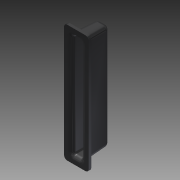
# Autodesk Inventor part: rubber-chamber
Saved by Autodesk Inventor 2015 (Build 190159000, 159)
## iProperties
Created: 2014-10-09
Part Number: rubber-chamber
Material: Rubber
Document SubType Name: Modeling
Designer: Adam
Density: 0.93 g/cm^3
Appearance: Rubber - Black - Version 1.1
Author: Adam
Autodesk Inventor part; units mm, degrees
ref_plane "YZ Plane" through (0, 0, 0) normal (1, 0, 0) x (0, 1, 0)
ref_plane "XZ Plane" through (0, 0, 0) normal (0, 1, 0) x (-1, 0, 0)
ref_plane "XY Plane" through (0, 0, 0) normal (0, 0, 1) x (1, 0, 0)
ref_plane "Work Plane1" through (0, 0, 0) normal (0, 0, 1) x (1, 0, 0)
sketch "Sketch1" plane through (0, 0, 0) normal (0, 0, 1) x (1, 0, 0)
  arc A0 (-28.0193, -5.5) -> (-30.0193, -3.5) centre (-30.0193, -5.5) ccw projected
  line L0 (-40.0193, -3.5) -> (-30.0193, -3.5) projected
  arc A1 (-40.0193, -3.5) -> (-42.0193, -5.5) centre (-40.0193, -5.5) ccw projected
  line L1 (-42.0193, -66.5) -> (-42.0193, -5.5) projected
  arc A2 (-42.0193, -66.5) -> (-40.0193, -68.5) centre (-40.0193, -66.5) ccw projected
  line L2 (-40.0193, -68.5) -> (-30.0193, -68.5) projected
  arc A3 (-30.0193, -68.5) -> (-28.0193, -66.5) centre (-30.0193, -66.5) ccw projected
  line L3 (-28.0193, -66.5) -> (-28.0193, -5.5) projected
  line L4 (-30.5193, -7.5) -> (-30.5193, -64.5) projected
  arc A4 (-32.0193, -66) -> (-30.5193, -64.5) centre (-32.0193, -64.5) ccw projected
  line L5 (-32.0193, -66) -> (-38.0193, -66) projected
  arc A5 (-39.5193, -64.5) -> (-38.0193, -66) centre (-38.0193, -64.5) ccw projected
  line L6 (-39.5193, -64.5) -> (-39.5193, -7.5) projected
  arc A6 (-38.0193, -6) -> (-39.5193, -7.5) centre (-38.0193, -7.5) ccw projected
  line L7 (-38.0193, -6) -> (-32.0193, -6) projected
  arc A7 (-30.5193, -7.5) -> (-32.0193, -6) centre (-32.0193, -7.5) ccw projected
  arc A8 (-28.3193, -5.5) -> (-30.0193, -3.8) centre (-30.0193, -5.5) ccw
  arc A9 (-40.0193, -3.8) -> (-41.7193, -5.5) centre (-40.0193, -5.5) ccw
  line L8 (-30.0193, -3.8) -> (-40.0193, -3.8)
  arc A10 (-30.0193, -68.2) -> (-28.3193, -66.5) centre (-30.0193, -66.5) ccw
  line L9 (-28.3193, -5.5) -> (-28.3193, -66.5)
  line L10 (-30.0193, -68.2) -> (-40.0193, -68.2)
  line L11 (-41.7193, -5.5) -> (-41.7193, -66.5)
  arc A11 (-41.7193, -66.5) -> (-40.0193, -68.2) centre (-40.0193, -66.5) ccw
  arc A12 (-31.0193, -7.5) -> (-32.0193, -6.5) centre (-32.0193, -7.5) ccw
  arc A13 (-38.0193, -6.5) -> (-39.0193, -7.5) centre (-38.0193, -7.5) ccw
  arc A14 (-32.0193, -65.5) -> (-31.0193, -64.5) centre (-32.0193, -64.5) ccw
  arc A15 (-39.0193, -64.5) -> (-38.0193, -65.5) centre (-38.0193, -64.5) ccw
  line L12 (-32.0193, -65.5) -> (-38.0193, -65.5)
  line L13 (-32.0193, -6.5) -> (-38.0193, -6.5)
  line L14 (-39.0193, -7.5) -> (-39.0193, -64.5)
  line L15 (-31.0193, -7.5) -> (-31.0193, -64.5)
  point P0 (0, 0)
  dimension "d0" = 0.3
  dimension "d1" = 0.5
  constraints: 17 point on circle, 16 end point, 14 tangent, 8 centre point, 8 coincident, 3 horizontal, 3 vertical, 2 parallel
  measures "d0" distance between parallel lines of L3 L9
  measures "d1" distance between parallel lines of L15 L4
extrude "Extrusion1" add sketch "Sketch1" along normal blind 1.5 contours L4 A4 L5 A5 L6 A6 L7 A7 | L9 A10 L10 A11 L11 A9 L8 A8
sketch "Sketch4" plane through (0, 0, 0) normal (0, 0, -1) x (-1, 0, 0)
  line L0 (31.0193, -64.5) -> (31.0193, -7.5) construction
  arc A0 (32.0193, -6.5) -> (31.0193, -7.5) centre (32.0193, -7.5) ccw construction
  line L1 (32.0193, -6.5) -> (38.0193, -6.5) construction
  arc A1 (39.0193, -7.5) -> (38.0193, -6.5) centre (38.0193, -7.5) ccw construction
  line L2 (39.0193, -7.5) -> (39.0193, -64.5) construction
  arc A2 (38.0193, -65.5) -> (39.0193, -64.5) centre (38.0193, -64.5) ccw construction
  line L3 (38.0193, -65.5) -> (32.0193, -65.5) construction
  arc A3 (31.0193, -64.5) -> (32.0193, -65.5) centre (32.0193, -64.5) ccw construction
  arc A4 (30.0193, -3.8) -> (28.3193, -5.5) centre (30.0193, -5.5) ccw construction
  line L4 (28.3193, -66.5) -> (28.3193, -5.5) construction
  arc A5 (28.3193, -66.5) -> (30.0193, -68.2) centre (30.0193, -66.5) ccw construction
  line L5 (40.0193, -68.2) -> (30.0193, -68.2) construction
  arc A6 (40.0193, -68.2) -> (41.7193, -66.5) centre (40.0193, -66.5) ccw construction
  line L6 (41.7193, -5.5) -> (41.7193, -66.5) construction
  arc A7 (41.7193, -5.5) -> (40.0193, -3.8) centre (40.0193, -5.5) ccw construction
  line L7 (30.0193, -3.8) -> (40.0193, -3.8) construction
  line L8 (37.5193, -8) -> (32.5193, -8)
  line L9 (32.5193, -8) -> (32.5193, -64)
  line L10 (32.5193, -64) -> (37.5193, -64)
  line L11 (37.5193, -64) -> (37.5193, -8)
  line L12 (31.0193, -6.5) -> (39.0193, -6.5)
  line L13 (39.0193, -6.5) -> (39.0193, -65.5)
  line L14 (39.0193, -65.5) -> (31.0193, -65.5)
  line L15 (31.0193, -65.5) -> (31.0193, -6.5)
  line L16 (31.0193, -64.5) -> (31.0193, -7.5) projected
  point P0 (0, 0)
  dimension "d4" = 1.5
  dimension "d5" = 1.5
  dimension "d6" = 1.5
  dimension "d7" = 1.5
  constraints: 16 end point, 4 collinear, 4 parallel, 2 horizontal, 2 perpendicular
  measures "d4" distance between parallel lines of L2 L11
  measures "d5" distance between parallel lines of L9 L0
  measures "d6" distance between parallel lines of L1 L8
  measures "d7" distance between parallel lines of L3 L10
extrude "Extrusion2" add sketch "Sketch4" along normal blind 12
sketch "Sketch5" plane through (0, 0, 0) normal (0, 0, 1) x (1, 0, 0)
  arc A0 (-32.0193, -65.5) -> (-31.0193, -64.5) centre (-32.0193, -64.5) ccw projected
  line L0 (-31.0193, -64.5) -> (-31.0193, -7.5) projected
  arc A1 (-31.0193, -7.5) -> (-32.0193, -6.5) centre (-32.0193, -7.5) ccw projected
  line L1 (-32.0193, -6.5) -> (-38.0193, -6.5) projected
  arc A2 (-38.0193, -6.5) -> (-39.0193, -7.5) centre (-38.0193, -7.5) ccw projected
  line L2 (-39.0193, -7.5) -> (-39.0193, -64.5) projected
  arc A3 (-39.0193, -64.5) -> (-38.0193, -65.5) centre (-38.0193, -64.5) ccw projected
  line L3 (-38.0193, -65.5) -> (-32.0193, -65.5) projected
  line L4 (-37.5193, -64) -> (-37.5193, -8) projected
  line L5 (-37.5193, -8) -> (-32.5193, -8) projected
  line L6 (-32.5193, -8) -> (-32.5193, -64) projected
  line L7 (-32.5193, -64) -> (-37.5193, -64) projected
  point P0 (0, 0)
extrude "Extrusion3" add sketch "Sketch5" along normal up to surface (1.5 mm away)
sketch "Sketch6" plane through (0, 0, -12) normal (0, 0, -1) x (-1, 0, 0)
  line L0 (37.5193, -8) -> (37.5193, -64) projected
  line L1 (37.5193, -64) -> (32.5193, -64) projected
  line L2 (32.5193, -64) -> (32.5193, -8) projected
  line L3 (32.5193, -8) -> (37.5193, -8) projected
  line L4 (39.0193, -6.5) -> (31.0193, -6.5) projected
  line L5 (31.0193, -6.5) -> (31.0193, -65.5) projected
  line L6 (31.0193, -65.5) -> (39.0193, -65.5) projected
  line L7 (39.0193, -65.5) -> (39.0193, -6.5) projected
  point P0 (0, 0)
extrude "Extrusion4" add sketch "Sketch6" along normal blind 1.5 contours L0 L1 L2 L3 | L7 L6 L5 L4
draft "FaceDraft1" angle 2.5 pull direction (0, 0, 1) faces at (-34.1859, -8, -3) (-32.5193, -26.6667, -3) (-37.5193, -26.6667, -3) (-34.1859, -64, -7.5) fixed edges at (-35.0193, -8, 1.5) (-32.5193, -36, 1.5) (-37.5193, -36, 1.5) (-35.0193, -64, -12)
draft "FaceDraft3" angle 2.5 pull direction (0, 0, -1) fixed plane through (-40.8193, -45.8333, 0) normal (0, 0, -1) faces at (-31.0193, -45.8333, -4.5) (-33.6859, -65.5, -4.5) (-39.0193, -45.8333, -4.5) (-33.6859, -6.5, -9)
fillet "Fillet3" radius 1 8 edges at (-35.0193, -8.5894, -12) (-37.2245, -64.2947, -5.25) (-36.9298, -36.2947, -12) (-35.0193, -64, -12) (-32.814, -64.2947, -5.25) (-33.1087, -36.2947, -12) (-32.814, -8.2947, -5.25) (-37.2245, -8.2947, -5.25)
fillet "Fillet4" radius 2.5 16 edges at (-38.4298, -36, -13.5) (-38.7245, -65.2053, -6.75) (-31.314, -65.2053, -6.75) (-35.0193, -64.9106, -13.5) (-31.6087, -36, -13.5) (-35.0193, -7.0894, -13.5) (-38.7245, -6.7947, -6.75) (-31.314, -6.7947, -6.75) (-37.2268, -64.2969, 1.5) (-35.0193, -64.5894, 1.5) (-32.8118, -64.2969, 1.5) (-32.5193, -36.2947, 1.5) (-32.8118, -8.2925, 1.5) (-35.0193, -8, 1.5) (-37.2268, -8.2925, 1.5) (-37.5193, -36.2947, 1.5)
fillet "Fillet5" radius 1 8 edges at (-35.0193, -6.5, 0) (-31.7505, -7.2312, 0) (-31.0193, -36, 0) (-31.7505, -64.7688, 0) (-35.0193, -65.5, 0) (-38.288, -64.7688, 0) (-39.0193, -36, 0) (-38.288, -7.2312, 0)
equation "\"d4\" = d2"
equation "\"d5\" = d2"
equation "\"d6\" = d2"
equation "\"d7\" = d2"
equation "\"d12\" = d2"
equation "\"d2\" = 1.5"
body "Solid1"
